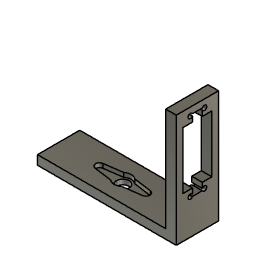
Connector v5 (Autodesk Fusion 360 design; units mm, degrees)
Autodesk Fusion 360 part; units mm, degrees
note: some values were not read from the file. Set by a fixed rule: which sketch regions a step uses.
sketch "base" plane through (0, 0, 0) normal (0, 0, 1) x (1, 0, 0)
  line L0 (53, -15) -> (-53, -15)
  line L1 (-53, -15) -> (-53, 15)
  line L2 (-53, 15) -> (53, 15)
  line L3 (53, 15) -> (53, -15)
  line L4 (53, -15) -> (-53, 15) construction
  line L5 (-53, -15) -> (53, 15) construction
  line L6 (53, -15) -> (45.5, -15)
  line L7 (45.5, -15) -> (45.5, 15)
  line L8 (45.5, 15) -> (53, 15)
  line L9 (53, 15) -> (53, -15)
  line L10 (0, 15) -> (0, -15)
  line L11 (-45.5, -15) -> (-45.5, 15)
  line L12 (-45.5, 15) -> (-53, 15)
  line L13 (-53, 15) -> (-53, -15)
  line L14 (-53, -15) -> (-45.5, -15)
  dimension "d1" = 106
  dimension "d2" = 30
  dimension "d3" = 7.5
  constraint horizontal L0
  constraint perpendicular L0 L1
  constraint parallel L0 L2
  constraint parallel L1 L3
  constraint coincident L4 origin
  constraint coincident L5 origin
  constraint horizontal L6
  constraint vertical L7
  constraint horizontal L8
  constraint vertical L9
  constraint midpoint L2 L10.start
  constraint midpoint L0 L10.end
  constraint coincident L2.end L8
  constraint symmetric L0.start L10 L0.end
  constraint symmetric L6.end L10 L11.start
  constraint symmetric L7.end L10 L11.end
  constraint symmetric L2.end L10 L1.end
  measures "d1" distance of L1.end L2.end
  measures "d2" distance of L0.end L1.end
  measures "d3" distance of L0.start L6.end
extrude "Extrude1" add sketch "base" along normal blind 6.5 contours L0 L2 L7 L10 | L0 L2 L10 L11
extrude "Extrude2" add sketch "base" along normal blind 80 contours L0 L2 L3 L6 L7 L8 L9
sketch "tilt holder" plane through (53, 0, 0) normal (1, 0, 0) x (0, 1, 0)
  line L0 (-15, 0) -> (15, 0)
  line L1 (15, 0) -> (15, 80)
  line L2 (15, 80) -> (-15, 80)
  line L3 (-15, 80) -> (-15, 0)
  line L4 (-10.25, 70) -> (10.25, 70)
  line L5 (10.25, 70) -> (10.25, 29.5)
  line L6 (10.25, 29.5) -> (-10.25, 29.5)
  line L7 (-10.25, 29.5) -> (-10.25, 70)
  line L8 (0, 80) -> (0, 0)
  dimension "d8" = 20.5
  dimension "d9" = 40.5
  dimension "d10" = 10
  constraint horizontal L4
  constraint vertical L5
  constraint horizontal L6
  constraint vertical L7
  constraint midpoint L2 L8.start
  constraint coincident L8.end origin
  measures "d8" distance of L4.start L4.end
  measures "d9" distance of L4.start L6.end
  measures "d10" distance of L2 L4
extrude "Extrude3" cut sketch "tilt holder" against normal blind 10 contours L4 L5 L6 L8 | L4 L6 L7 L8
sketch "screw holes" plane through (53, 0, 0) normal (1, 0, 0) x (0, 1, 0)
  line L0 (10.25, 70) -> (10.25, 29.5)
  line L1 (10.25, 29.5) -> (-10.25, 29.5)
  line L2 (-10.25, 29.5) -> (-10.25, 70)
  line L3 (-10.25, 70) -> (10.25, 70)
  line L4 (-15, 0) -> (15, 0)
  line L5 (15, 0) -> (15, 80)
  line L6 (15, 80) -> (-15, 80)
  line L7 (-15, 80) -> (-15, 0)
  line L8 (0, 80) -> (0, 0)
  circle A0 centre (5, 74.496) radius 1.675
  circle A1 centre (-5, 74.496) radius 1.675
  line L9 (10.25, 49.75) -> (-10.25, 49.75)
  circle A2 centre (-5, 25.004) radius 1.675
  circle A3 centre (5, 25.004) radius 1.675
  dimension "d13" = 3.35
  dimension "d14" = 10
  dimension "d15" = 4.496
  constraint midpoint L6 L8.start
  constraint coincident L8.end origin
  constraint symmetric L8 A0 A1
  constraint midpoint L0 L9.start
  constraint midpoint L2 L9.end
  constraint symmetric A0 L9 A3
  constraint symmetric A1 L9 A2
  measures "d13" diameter of A0
  measures "d14" distance of A0.centre A1.centre
  measures "d15" distance of L3 A0.centre
extrude "Extrude4" cut sketch "screw holes" against normal blind 15 contours A0 | A1 | A2 | A3
sketch "pan indent" plane through (0, 0, 6.5) normal (0, 0, 1) x (-1, 0, 0)
  line L0 (-45.5, 15) -> (-45.5, -15)
  line L1 (-45.5, -15) -> (45.5, -15)
  line L2 (45.5, 15) -> (-45.5, 15)
  line L3 (45.5, -15) -> (45.5, 15)
  line L4 (45.5, 0) -> (-45.5, 0)
  line L5 (0, -15) -> (0, 15)
  line L6 (3.969, -4.6322) -> (16.8952, -2.8225)
  arc A0 (3.969, 4.6322) -> (-3.969, 4.6322) centre (0, 0) ccw
  line L7 (16.8952, 2.8225) -> (3.969, 4.6322)
  line L8 (-16.8952, -2.8225) -> (-3.969, -4.6322)
  circle A1 centre (0, 0) radius 4.55
  arc A2 (-16.8952, 2.8225) -> (-16.8952, -2.8225) centre (-16.5, 0) ccw
  arc A3 (-3.969, -4.6322) -> (3.969, -4.6322) centre (0, 0) ccw
  arc A4 (16.8952, -2.8225) -> (16.8952, 2.8225) centre (16.5, 0) ccw
  line L9 (-16.8952, 2.8225) -> (-3.969, 4.6322)
  point P0 (0, 6.1)
  dimension "d51" = 9.1
  dimension "d52" = 6.1
  dimension "d53" = 2.85
  dimension "d54" = 33.7903
  dimension "d55" = 12.9262
  dimension "d56" = 7.938
  constraint midpoint L3 L4.start
  constraint midpoint L0 L4.end
  constraint midpoint L1 L5.start
  constraint midpoint L2 L5.end
  constraint tangent L8 A2
  constraint tangent L7 A4
  constraint tangent L6 A4
  constraint coincident L4 A4.centre
  constraint coincident L4 A2.centre
  constraint coincident L4 A0.centre
  constraint coincident L5 A0.centre
  constraint symmetric L4 A0 A3
  constraint symmetric L5 A2 A4
  constraint midpoint A0 P0
  constraint coincident L5 P0
  constraint vertical L6.start A0.start
  constraint vertical A2.start L8.start
  constraint symmetric L4 L8.start A2.start
  constraint symmetric L4 L8.end A0.end
  measures "d51" diameter of A1
  measures "d52" radius of A3
  measures "d53" radius of A2
  measures "d54" distance of L6.end L8.start
  measures "d55" horizontal distance of L8.start L8.end
  measures "d56" distance of A0.start A0.end
extrude "Extrude9" cut sketch "pan indent" against normal blind 3 contours L4 L5 A0 A1 A2 L9 | L4 L5 L8 A1 A2 A3 | L4 L5 A0 L7 A1 A4 | L4 L5 L6 A1 A3 A4
extrude "Extrude10" cut 1 faces at (-0.7414, -1.5395, 6.5) along direction (0, 0, -1) blind 15
sketch "wire room" plane through (53, 0, 0) normal (1, 0, 0) x (0, 1, 0)
  circle A0 centre (5, 74.496) radius 1.675
  circle A1 centre (-5, 25.004) radius 1.675
  circle A2 centre (-5, 74.496) radius 1.675
  circle A3 centre (5, 25.004) radius 1.675
  line L0 (10.25, 70) -> (10.25, 29.5)
  line L1 (10.25, 29.5) -> (-10.25, 29.5)
  line L2 (-10.25, 29.5) -> (-10.25, 70)
  line L3 (-10.25, 70) -> (10.25, 70)
  line L4 (-15, 0) -> (15, 0)
  line L5 (15, 0) -> (15, 80)
  line L6 (15, 80) -> (-15, 80)
  line L7 (-15, 80) -> (-15, 0)
  line L8 (-10.25, 70) -> (-10.25, 29.5) construction
  line L9 (-10.25, 49.75) -> (10.25, 49.75)
  line L10 (-3.4739, 24.3135) -> (3.4739, 24.3135)
  line L11 (3.4739, 24.3135) -> (3.4739, 29.5)
  line L12 (-3.4739, 24.3135) -> (-3.4739, 29.5)
  line L13 (-3.4739, 75.1865) -> (-3.4739, 70)
  line L14 (-3.4739, 75.1865) -> (3.4739, 75.1865)
  line L15 (3.4739, 75.1865) -> (3.4739, 70)
  dimension "d66" = 6.9479
  constraint coincident L2.end L3.start
  constraint coincident L1.end L2.start
  constraint midpoint L8 L9.start
  constraint midpoint L0 L9.end
  constraint coincident A1 L10.start
  constraint coincident A3 L10.end
  constraint parallel L1 L10
  constraint coincident L1 L11.end
  constraint perpendicular L1 L11
  constraint coincident L1 L12.end
  constraint perpendicular L1 L12
  constraint symmetric L9 L10.start L13.start
  constraint symmetric L9 L10.end L14.end
  constraint symmetric L9 L11.end L15.end
  constraint symmetric L9 L12.end L13.end
  measures "d66" distance of L10.start L10.end
extrude "Extrude11" cut sketch "wire room" against normal blind 10 contours A0 A2 L3 L13 L14 L15 | A1 A3 L1 L10 L11 L12
